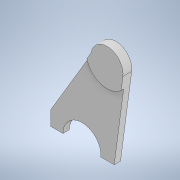
# Autodesk Inventor part: volante conjunto
Saved by Autodesk Inventor 2022.1 (Build 261234020, 234B)
## iProperties
Created: 2023-08-18
Part Number: volante conjunto
Material: Generic
Document SubType Name: Modeling
Designer: SENAI
Density: 1 g/cm^3
Appearance: Default
Author: SENAI
Autodesk Inventor part; units mm, degrees
ref_plane "YZ Plane" through (0, 0, 0) normal (1, 0, 0) x (0, 1, 0)
ref_plane "XZ Plane" through (0, 0, 0) normal (0, 1, 0) x (-1, 0, 0)
ref_plane "XY Plane" through (0, 0, 0) normal (0, 0, 1) x (1, 0, 0)
sketch "Sketch1" plane through (0, 0, 0) normal (0, 0, 1) x (1, 0, 0)
  line L0 (0, 0) -> (30, 0)
  arc A0 (122.3584, -3.6921) -> (30, 0) centre (76.2499, -0.076) ccw
  line L1 (122.3584, -3.6921) -> (154.7584, -3.6921)
  line L2 (154.7584, -3.6921) -> (357.7584, -3.6921) construction
  line L3 (0, 0) -> (0, 35)
  arc A1 (181.6354, 197.5208) -> (104.7506, 210.6385) centre (143.2612, 204.4794) ccw
  line L4 (122.3584, -3.6921) -> (132.3584, -3.6921)
  line L5 (0, 35) -> (104.7506, 210.6385)
  line L6 (154.7584, -3.6921) -> (181.9168, 199.3079)
  dimension "d0" = 30
  dimension "d1" = 92.5
  dimension "d2" = 32.4
  dimension "d3" = 203
  dimension "d5" = 35
  dimension "d7" = 10
  dimension "d9" = 78
  dimension "d10" = 203
  constraints: 14 end point, 5 point on circle, 3 horizontal, 2 centre point, 1 point on line, 1 tangent, 1 vertical
  measures "d0" distance of L0.start L0.end
  measures "d1" diameter of A0
  measures "d2" distance of L1.start L1.end
  measures "d3" distance of L1.end A1.start
  measures "d5" distance of L0.start L3.end
  measures "d7" distance of L1.start L4.end
  measures "d9" diameter of A1
  measures "d10" vertical distance of L1.end L6.end
sketch "Sketch2" plane through (0, 0, 0) normal (0, 0, 1) x (1, 0, 0)
  point P0 (0, 0)
extrude "Extrusion1" add sketch "Sketch1" along normal blind 15.3
sketch "Sketch3" plane through (0, 0, 15.3) normal (0, 0, 1) x (1, 0, 0)
  line L0 (154.7584, -3.6921) -> (181.9168, 199.3079) projected
  arc A0 (94.1987, 192.9457) -> (177.6835, 167.6655) centre (143.2612, 204.4794) ccw
  arc A1 (181.9168, 199.3079) -> (104.7506, 210.6385) centre (143.2612, 204.4794) ccw projected
  line L1 (104.7506, 210.6385) -> (94.1987, 192.9457)
  line L2 (104.7506, 210.6385) -> (0, 35) projected
  line L3 (181.9168, 199.3079) -> (177.6835, 167.6655)
  arc A2 (181.9168, 199.3079) -> (104.7506, 210.6385) centre (143.2612, 204.4794) ccw
  point P0 (0, 0)
  dimension "d19" = 100.8
  constraints: 4 end point, 4 point on circle, 2 centre point, 2 point on line, 2 tangent
  measures "d19" diameter of A0
extrude "Extrusion2" add sketch "Sketch3" along normal blind 6
body "Solid1"
